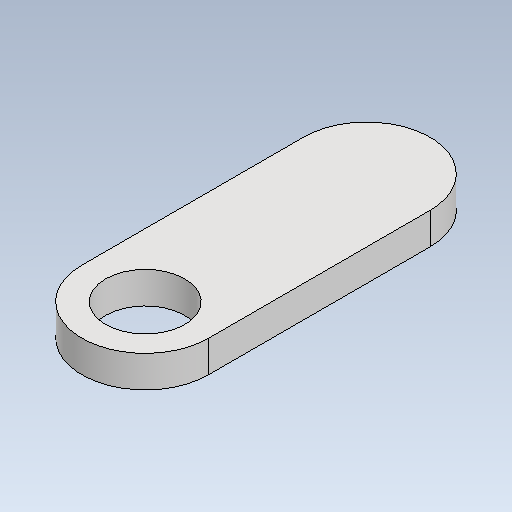
# Autodesk Inventor part: servo-arm
Saved by Autodesk Inventor 2025 (Build 290162000, 162)
## iProperties
Created: 2025-08-20
Part Number: servo-arm
Material: Generic
Document SubType Name: Modeling
Designer: HP
Density: 1 g/cm^3
Appearance: Default
Author: HP
Autodesk Inventor part; units mm, degrees
ref_plane "YZ Plane" through (0, 0, 0) normal (1, 0, 0) x (0, 1, 0)
ref_plane "XZ Plane" through (0, 0, 0) normal (0, 1, 0) x (-1, 0, 0)
ref_plane "XY Plane" through (0, 0, 0) normal (0, 0, 1) x (1, 0, 0)
sketch "Sketch1" plane through (0, 0, 0) normal (0, 1, 0) x (-1, 0, 0)
  line L0 (0, 7) -> (0, -7) construction
  line L1 (-4, 7) -> (-4, -7)
  line L2 (4, -7) -> (4, 7)
  arc A0 (4, 7) -> (-4, 7) centre (0, 7) ccw
  arc A1 (-4, -7) -> (4, -7) centre (0, -7) ccw
  circle A2 centre (0, 7) radius 2.5
  point P0 (0, 0)
  point P1 (0, 0)
  point P2 (0, -11)
  dimension "d0" = 8
  dimension "d1" = 18
  dimension "d2" = 5
  constraints: 8 end point, 5 point on circle, 4 tangent, 3 centre point, 2 coincident, 1 midpoint, 1 parallel, 1 vertical
  measures "d0" distance between parallel lines of L1 L2
  measures "d1" distance of point (0, -11) L0.start
  measures "d2" diameter of A2
extrude "Extrusion1" add sketch "Sketch1" along normal blind 2
body "Solid1"
